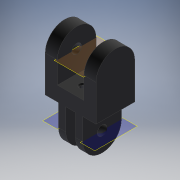
# Autodesk Inventor part: Falange-media2
Saved by Autodesk Inventor 2018 (Build 220112000, 112)
## iProperties
Created: 2017-06-03
Part Number: Falange-media2
Material: Genérico
Document SubType Name: Modeling
Designer: Vitor
Density: 1 g/cm^3
Appearance: Padrão
Author: Vitor
Autodesk Inventor part; units mm, degrees
ref_plane "YZ Plane" through (0, 0, 0) normal (1, 0, 0) x (0, 1, 0)
ref_plane "XZ Plane" through (0, 0, 0) normal (0, 1, 0) x (-1, 0, 0)
ref_plane "XY Plane" through (0, 0, 0) normal (0, 0, 1) x (1, 0, 0)
sketch "Esboço14" plane through (0, 0, 0) normal (0, 0, 1) x (1, 0, 0)
  line L0 (0, 0) -> (21, 0)
  line L1 (21, 0) -> (21, -16)
  line L2 (21, -16) -> (0, -16)
  line L3 (0, -16) -> (0, 0)
  dimension "d47" = 21
  dimension "d48" = 16
  constraints: 8 end point, 2 parallel, 1 horizontal, 1 perpendicular
  measures "d47" distance of L1.end L2.end
  measures "d48" distance of L0.end L1.end
extrude "Extrusão14" add sketch "Esboço14" along normal blind 6
sketch "Esboço15" plane through (21, -16, 0) normal (1, 0, 0) x (0, 0, -1)
  line L0 (-6, 16) -> (-15, 16)
  line L1 (-15, 16) -> (-15, 0)
  line L2 (-15, 0) -> (-6, 0)
  line L3 (-6, 16) -> (-6, 0) projected
  line L4 (-6, 0) -> (-6, 16)
  circle A0 centre (-15, 8) radius 8
  point P0 (0, 16)
  dimension "d51" = 9
  dimension "d52" = 16
  constraints: 8 end point, 2 perpendicular, 1 collinear, 1 horizontal, 1 midpoint, 1 vertical alignment, 2 other
  measures "d51" distance of L0.start L0.end
  measures "d52" distance of L0.end L1.end
extrude "Extrusão15" add sketch "Esboço15" against normal blind 5
sketch "Esboço16" plane through (0, -16, 0) normal (-1, 0, 0) x (0, 0, 1)
  line L0 (6, 16) -> (6, 0) projected
  line L1 (0, 16) -> (15, 16) projected
  line L2 (6, 16) -> (15, 16)
  arc A0 (15, 0) -> (15, 16) centre (15, 8) ccw projected
  line L3 (15, 16) -> (15, 0)
  line L4 (15, 0) -> (6, 0)
  line L5 (6, 0) -> (6, 16)
  circle A1 centre (15, 8) radius 8
  constraints: 8 end point, 3 perpendicular, 1 coincident, 1 collinear, 1 tangent, 1 vertical alignment, 2 other
extrude "Extrusão16" add sketch "Esboço16" against normal blind 5
sketch "Esboço17" plane through (0, 0, 0) normal (0, 0, -1) x (-1, 0, 0)
  line L0 (-16, 0) -> (-5, 0) projected
  line L1 (-10.5, 0) -> (-10.5, -16)
  line L2 (-21, -16) -> (0, -16) projected
  line L3 (-10.5, -16) -> (-8.5, -16)
  line L4 (-8.5, -16) -> (-8.5, 0)
  line L5 (-8.5, 0) -> (-12.5, 0)
  line L6 (-12.5, 0) -> (-12.5, -16)
  line L7 (-15.5, -8) -> (-15.5, -6)
  line L8 (-15.5, -8) -> (-13.5, -8) construction
  line L9 (-15.5, -6) -> (-8.5, -6)
  line L10 (-8.5, -6) -> (-5.5, -6)
  line L11 (-5.5, -6) -> (-5.5, -10)
  line L12 (-5.5, -10) -> (-15.5, -10)
  line L13 (-15.5, -10) -> (-15.5, -8)
  line L14 (-15.5, -6) -> (-12.5, -6)
  line L15 (-12.5, -10) -> (-12.5, -6)
  line L16 (-8.5, -6) -> (-8.5, -10)
  point P0 (0, 0)
  dimension "d57" = 2
  dimension "d58" = 4
  dimension "d60" = 2
  dimension "d61" = 90
  dimension "d62" = 3
  dimension "d63" = 4
  constraints: 30 end point, 10 point on line, 9 perpendicular, 2 midpoint, 1 collinear, 1 horizontal, 1 vertical
  measures "d57" distance of L1.end L3.end
  measures "d58" distance of L4.end L5.end
  measures "d60" distance of L7.start L7.end
  measures "d61" angle of L8 L7
  measures "d62" distance of L9.end L10.end
  measures "d63" distance of L10.end L11.end
extrude "Extrusão17" add sketch "Esboço17" along normal blind 9 contours L9 L1 L12 L6 | L6 L12 L13 L7 L9 | L9 L4 L12 L1 | L10 L11 L12 L4
sketch "Esboço18" plane through (5.5, -10, 0) normal (-1, 0, 0) x (0, 0, 1)
  line L0 (-9, 0) -> (-9, 4) projected
  circle A0 centre (-9, 2) radius 8
  line L1 (-9, 10) -> (0, 10)
  line L2 (0, -6) -> (0, 10) projected
  line L3 (0, 10) -> (0, -6)
  line L4 (0, -6) -> (-9, -6)
  dimension "d66" = 16
  constraints: 6 end point, 2 point on circle, 1 centre point, 1 midpoint, 1 perpendicular, 1 tangent
  measures "d66" diameter of A0
extrude "Extrusão18" add sketch "Esboço18" against normal blind 3
sketch "Esboço19" plane through (15.5, -10, 0) normal (1, 0, 0) x (0, 0, -1)
  line L0 (9, 4) -> (9, 0) projected
  circle A0 centre (9, 2) radius 8
  line L1 (0, 10) -> (9, 10) projected
  line L2 (9, 10) -> (0, 10)
  line L3 (0, 10) -> (0, -6) projected
  line L4 (0, 10) -> (0, -6)
  line L5 (9, -6) -> (0, -6) projected
  line L6 (0, -6) -> (9, -6)
  constraints: 6 end point, 3 collinear, 1 centre point, 1 midpoint, 1 point on circle, 1 point on line
extrude "Extrusão19" add sketch "Esboço19" against normal blind 3
fillet "Arredondamento6" radius 2 2 edges at (10.5, -6, -9) (10.5, -10, -9)
sketch "Esboço20" plane through (0, 0, 0) normal (0, 0, -1) x (-1, 0, 0)
  line L0 (-8.5, -10) -> (-12.5, -10) projected
  line L1 (-10.5, -10) -> (-10.5, -11)
  line L2 (-8.5, -6) -> (-12.5, -6) projected
  line L3 (-10.5, -6) -> (-10.5, -5)
  circle A0 centre (-10.5, -5) radius 1
  circle A1 centre (-10.5, -11) radius 1
  point P0 (0, 0)
  dimension "d72" = 1
  dimension "d73" = 1
  dimension "d74" = 2
  dimension "d75" = 2
  constraints: 4 end point, 2 centre point, 2 coincident, 2 midpoint, 2 vertical
  measures "d72" distance of L1.start L1.end
  measures "d73" distance of L3.start L3.end
  measures "d74" diameter of A0
  measures "d75" diameter of A1
extrude "Extrusão20" cut sketch "Esboço20" against normal blind 8
chamfer "Chanfro1" distance 0.5 angle 45 2 edges at (11.5, -5, 6) (11.5, -11, 6)
fillet "Arredondamento7" radius 0.5 4 edges at (11.2071, -4.2929, 0) (9.7929, -5.7071, 0) (11.2071, -11.7071, 0) (9.7929, -10.2929, 0)
ref_plane "Plano de trabalho1" through (0, 0, -9) normal (0, 0, -1) x (-1, 0, 0)
sketch "Esboço21" plane through (0, 0, -9) normal (0, 0, -1) x (-1, 0, 0)
  line L0 (-15.5, -16) -> (-15.5, 0) projected
  line L1 (-15.5, -8) -> (-16.5, -8)
  line L2 (-15.5, -8) -> (-15.5, -10)
  arc A0 (-16.5, -8) -> (-15.5, -10) centre (-14.5168, -8.2584) ccw
  point P0 (0, 0)
  dimension "d83" = 1
  dimension "d84" = 2
  dimension "d85" = 2
  constraints: 4 end point, 2 point on circle, 1 centre point, 1 horizontal, 1 midpoint, 1 point on line
  measures "d83" distance of L1.start L1.end
  measures "d84" distance of L1.start L2.end
  measures "d85" radius of A0
revolve "Revolução1" add sketch "Esboço21" angle 360 about axis through (15.5, -8, -9) along (1, 0, 0)
ref_plane "Plano de trabalho2" through (0, 0, -9) normal (0, 0, -1) x (-1, 0, 0)
sketch "Esboço22" plane through (0, 0, -9) normal (0, 0, -1) x (-1, 0, 0)
  line L0 (-5.5, 0) -> (-5.5, -16) projected
  line L1 (-5.5, -8) -> (-4.5, -8)
  line L2 (-5.5, -8) -> (-5.5, -6)
  arc A0 (-4.5, -8) -> (-5.5, -6) centre (-6.4832, -7.7416) ccw
  point P0 (0, 0)
  dimension "d88" = 1
  dimension "d89" = 2
  dimension "d90" = 2
  constraints: 4 end point, 2 point on circle, 1 centre point, 1 horizontal, 1 midpoint, 1 point on line
  measures "d88" distance of L1.start L1.end
  measures "d89" distance of L1.start L2.end
  measures "d90" radius of A0
revolve "Revolução2" add sketch "Esboço22" angle 360 about axis through (5.5, -8, -9) along (-1, 0, 0)
ref_plane "Plano de trabalho3" through (0, 0, 15) normal (0, 0, 1) x (1, 0, 0)
sketch "Esboço23" plane through (0, 0, 15) normal (0, 0, 1) x (1, 0, 0)
  line L0 (16, -16) -> (16, 0) projected
  line L1 (16, -8) -> (17, -8)
  line L2 (16, -8) -> (16, -10)
  line L3 (5, 0) -> (5, -16) projected
  line L4 (5, -8) -> (4, -8)
  line L5 (5, -8) -> (5, -6)
  arc A0 (5, -6) -> (4, -8) centre (5.9832, -7.7416) ccw
  arc A1 (16, -10) -> (17, -8) centre (15.0168, -8.2584) ccw
  point P0 (0, 0)
  dimension "d93" = 1
  dimension "d94" = 2
  dimension "d95" = 1
  dimension "d96" = 2
  dimension "d97" = 2
  dimension "d98" = 2
  constraints: 8 end point, 4 point on circle, 2 centre point, 2 horizontal, 2 midpoint, 2 point on line
  measures "d93" distance of L1.start L1.end
  measures "d94" distance of L1.start L2.end
  measures "d95" distance of L4.start L4.end
  measures "d96" distance of L4.start L5.end
  measures "d97" radius of A0
  measures "d98" radius of A1
revolve "Revolução3" cut sketch "Esboço23" angle 360 about axis through (16, -8, 15) along (1, 0, 0)
